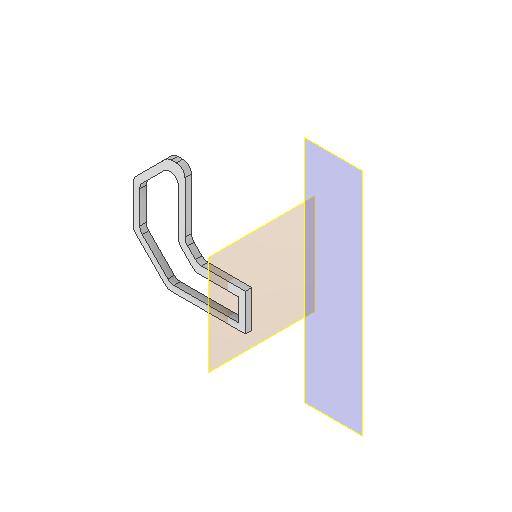
# Autodesk Inventor part: Matchboxscope_Lightperiscope_long_V0
Saved by Autodesk Inventor 2022 (Build 260153000, 153)
## iProperties
Created: 2022-03-26
Part Number: Matchboxscope_Lightperiscope_long_V0
Material: Generic
Document SubType Name: Modeling
Designer: Prakash Lab
Density: 1 g/cm^3
Appearance: Default
Author: Prakash Lab
Autodesk Inventor part; units mm, degrees
ref_plane "YZ Plane" through (0, 0, 0) normal (1, 0, 0) x (0, 1, 0)
ref_plane "XZ Plane" through (0, 0, 0) normal (0, 1, 0) x (-1, 0, 0)
ref_plane "XY Plane" through (0, 0, 0) normal (0, 0, 1) x (1, 0, 0)
ref_plane "Work Plane1" through (118.9518, 9.9874, -13.1749) normal (0.4728584, -0.8811384, 0) x (0, 0, -1)
sketch "Sketch1" plane through (118.9518, 9.9874, -13.1749) normal (0.4728584, -0.8811384, 0) x (0, 0, -1)
  line L0 (-16.5984, 5.5392) -> (-16.5984, 5.9228)
  line L1 (-1.2281, -14.4596) -> (-31.7652, -14.4596) construction
  line L2 (-16.5984, 11.5008) -> (-16.5984, -0.9971) projected
  line L3 (-15.5984, -2) -> (-12.5984, -2)
  line L4 (-16.5984, 2) -> (-12.5984, 2)
  line L5 (-16.5984, -2.6601) -> (-27.5984, -2.6601)
  line L6 (-27.5984, -2.6601) -> (-30.5984, -5.6601)
  line L7 (-30.5984, -5.6601) -> (-30.5984, -8.4596)
  line L8 (-30.5984, -8.4596) -> (-30.5984, -20.4596)
  line L9 (-30.5984, -20.4596) -> (-34.5984, -20.4596)
  line L10 (-34.5984, -20.4596) -> (-42.5984, -12.4596)
  line L11 (-42.5984, -12.4596) -> (-42.5984, -2.0772)
  line L12 (-42.5984, -2.0772) -> (-34.5984, 5.9228)
  line L13 (-34.5984, 5.9228) -> (-16.5984, 5.9228)
  line L14 (-16.5984, 0.8574) -> (-16.5984, 5.9228)
  line L15 (-16.5984, 3.3399) -> (-48.439, 3.3399) construction
  line L16 (-16.5984, -0.9971) -> (-16.5984, -2.6601)
  line L17 (-16.5984, -0.0772) -> (-40.5984, -0.0772) construction
  line L18 (-40.5984, -0.0772) -> (-40.5984, -14.4596) construction
  line L19 (-16.5984, -0.0772) -> (-40.5984, -0.0772)
  line L20 (-19.5984, -2.6601) -> (-17.0984, -2.6601) projected
  point P0 (-13.1749, -109.5356)
  point P1 (-16.5984, 0.8574)
  dimension "d25" = 135
  dimension "d26" = 4
  dimension "d27" = 6
  dimension "d28" = 2.5829
  dimension "d29" = 6
  dimension "d31" = 12
  dimension "d40" = 3
  dimension "d42" = 26
  dimension "d45" = 0
  dimension "d50" = 8
  dimension "d62" = 0
  constraints: 38 end point, 7 point on line, 6 horizontal, 5 perpendicular, 4 collinear, 2 parallel, 4 other
  measures "d25" angle of L9 L10
  measures "d26" distance between parallel lines of L4 L3
  measures "d27" distance between parallel lines of L5 L15
  measures "d28" distance between parallel lines of L13 L15
  measures "d29" distance between parallel lines of L9 L1
  measures "d31" distance between parallel lines of L7 L11
  measures "d40" horizontal distance of L5.end L6.end
  measures "d42" distance between parallel lines of L16 L11
  measures "d45" horizontal distance of L12.end L9.end
  measures "d50" distance from line of L9.end L11
  measures "d62" distance between parallel lines of L20 L5
extrude "Extrusion1" add sketch "Sketch1" along normal blind 1.5
sketch "Sketch2" plane through (119.6611, 8.6657, -13.1749) normal (0.4728584, -0.8811384, 0) x (0.8811384, 0.4728584, 0)
  line L0 (-2.0772, 42.5984) -> (-12.4596, 42.5984) projected
  line L1 (-12.4596, 42.5984) -> (-20.4596, 34.5984) projected
  line L2 (-20.4596, 34.5984) -> (-20.4596, 30.5984) projected
  line L3 (-20.4596, 30.5984) -> (-5.6601, 30.5984) projected
  line L4 (-5.6601, 30.5984) -> (-2.6601, 27.5984) projected
  line L5 (-2.6601, 27.5984) -> (-2.6601, 16.5984) projected
  line L6 (5.9228, 16.5984) -> (5.9228, 34.5984) projected
  line L7 (5.9228, 34.5984) -> (-2.0772, 42.5984) projected
  line L8 (-2.6601, 16.5984) -> (5.9228, 16.5984) projected
  line L9 (-11.8383, 41.0984) -> (-2.6985, 41.0984)
  line L10 (-2.6985, 41.0984) -> (4.4228, 33.9771)
  line L11 (4.4228, 33.9771) -> (4.4228, 18.0984)
  line L12 (4.4228, 18.0984) -> (-0.9902, 18.0984)
  line L13 (-0.9902, 18.0984) -> (-1.1601, 18.0962)
  line L14 (-1.1601, 18.0962) -> (-1.1601, 28.2197)
  line L15 (-1.1601, 28.2197) -> (-5.0388, 32.0984)
  line L16 (-5.0388, 32.0984) -> (-8.9884, 32.0984)
  line L17 (-8.9884, 32.0984) -> (-9.9596, 32.0984)
  line L18 (-9.9596, 32.0984) -> (-18.9596, 32.0984)
  line L19 (-18.9596, 32.0984) -> (-18.9596, 33.9771)
  line L20 (-18.9596, 33.9771) -> (-11.8383, 41.0984)
  point P0 (-109.5356, 13.1749)
  point P1 (-0.7471, 18.0984)
  dimension "d41" = 1.5
  dimension "d63" = 1.5
  constraints: 24 end point, 1 horizontal, 6 other
  measures "d41" distance between parallel lines of L0 L9
  measures "d63" distance between parallel lines of L3 L18
extrude "Extrusion2" [suppressed]
sketch "Sketch3" plane through (103.5006, 1.6956, 17.4235) normal (0, 0, -1) x (-0.8811384, -0.4728584, 0)
  circle A0 centre (-2.8052, -7.75) radius 4.5
  line L0 (3.1948, 0) -> (-8.8052, 0) projected
  line L1 (-8.8052, 0) -> (-8.8052, -15.5) projected
  line L2 (3.1948, -15.5) -> (-8.8052, -15.5) projected
  line L3 (3.1948, 0) -> (3.1948, -15.5) projected
  point P0 (92.0001, 47.4471)
  constraints: 1 centre point
extrude "Extrusion3" cut sketch "Sketch3" against normal blind 1.5 contours A0
sketch "Sketch8" plane through (119.7213, 8.698, 3.4235) normal (0, 0, 1) x (0.8811384, 0.4728584, 0)
  circle A0 centre (-19.1075, 3.6497) radius 1.4001 projected
  circle A1 centre (-14.1578, 7.8923) radius 2 projected
  circle A2 centre (-14.1578, 7.8923) radius 3.3708
  point P0 (-109.604, 48.9471)
  constraints: 1 centre point
extrude "Extrusion8" cut sketch "Sketch8" along normal mid plane 14 contours A1 | A2
sketch "Sketch9" plane through (118.7885, 8.1974, 4.9235) normal (0, 0, 1) x (0.8811384, 0.4728584, 0)
  circle A0 centre (0.9902, -6.25) radius 1.352 projected
  circle A1 centre (0.9902, -6.25) radius 2.6601
  point P0 (-108.5454, 48.9471)
  constraints: 1 centre point, 1 coincident
extrude "Extrusion9" [suppressed]
ref_plane "Arbeitsebene3" through (124.1706, 12.788, 7.4235) normal (0, 0, -1) x (-0.8811384, -0.4728584, 0)
sketch "Skizze13" plane through (124.1706, 12.788, 7.4235) normal (0, 0, -1) x (-0.8811384, -0.4728584, 0)
  line L0 (0, 0) -> (0, -1.5) projected
  circle A0 centre (-2.8278, -9.3645) radius 1.1933 projected
  line L1 (8.5829, 0) -> (0, 0) projected
  line L2 (0, 0) -> (0, -15.5)
  line L3 (0, -15.5) -> (-6.5, -15.5)
  line L4 (-6.5, -15.5) -> (-6.5, 0)
  line L5 (-6.5, 0) -> (0, 0)
  circle A1 centre (-2.8278, -9.3645) radius 1.6 projected
  circle A2 centre (-2.8278, -9.3645) radius 1.75
  point P0 (115.4584, 47.4471)
  point P1 (-2.8531, -15.3156)
  dimension "d58" = 6.5
  dimension "d66" = 3.5
  constraints: 8 end point, 2 parallel, 1 centre point, 1 coincident, 1 perpendicular, 1 vertical, 1 other
  measures "d58" distance of L3.end L2.end
  measures "d66" diameter of A2
extrude "Extrusion13" [suppressed]
fillet "Rundung1" radius 2 7 edges at (124.5253, 12.1272, 21.4235) (108.3278, 3.4349, 29.4235) (101.2787, -0.348, 21.4235) (101.2787, -0.348, 17.4235) (114.3191, 6.6501, 17.4235) (116.9625, 8.0687, 14.4235) (117.4762, 8.3443, 29.4235)
sketch "Skizze14" plane through (118.9518, 9.9874, -13.1749) normal (-0.4728584, 0.8811384, 0) x (0.8811384, 0.4728584, 0)
  arc A0 (3.8371, -34.5629) -> (4.4228, -33.1487) centre (2.4228, -33.1487) ccw projected
  line L0 (3.8371, -34.5629) -> (-2.1127, -40.5126) projected
  arc A1 (-3.5269, -41.0984) -> (-2.1127, -40.5126) centre (-3.5269, -39.0984) ccw projected
  line L1 (-3.5269, -41.0984) -> (-11.0098, -41.0984) projected
  arc A2 (-12.4241, -40.5126) -> (-11.0098, -41.0984) centre (-11.0098, -39.0984) ccw projected
  line L2 (-12.4241, -40.5126) -> (-17.4241, -35.5126) projected
  arc A3 (-16.0098, -32.0984) -> (-17.4241, -35.5126) centre (-16.0098, -34.0984) ccw projected
  line L3 (-16.0098, -32.0984) -> (-5.4542, -32.0984) projected
  arc A4 (-5.4542, -32.0984) -> (-4.04, -31.5126) centre (-5.4542, -30.0984) ccw projected
  line L4 (-4.04, -31.5126) -> (-1.3329, -28.8055) projected
  arc A5 (-1.3329, -28.8055) -> (-0.7471, -27.3913) centre (-2.7471, -27.3913) ccw projected
  line L5 (-0.7471, -27.3913) -> (-0.7471, -18.0984) projected
  line L6 (-0.7471, -18.0984) -> (4.4228, -18.0984) projected
  line L7 (4.4228, -18.0984) -> (4.4228, -33.1487) projected
  point P0 (-109.5356, -13.1749)
extrude "Extrusion14" cut sketch "Skizze14" against normal blind 10
body "Solid1"
